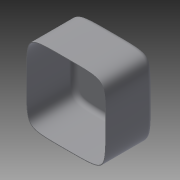
# Autodesk Inventor part: Base Plate
Saved by Autodesk Inventor 2014 SP1 (Build 180222100, 222)
## iProperties
Created: 2014-01-02
Part Number: Base Plate
Material: Generic
Document SubType Name: Modeling
Designer: tom
Density: 1 g/cm^3
Appearance: Default
Author: tom
Autodesk Inventor part; units mm, degrees
ref_plane "YZ Plane" through (0, 0, 0) normal (1, 0, 0) x (0, 1, 0)
ref_plane "XZ Plane" through (0, 0, 0) normal (0, 1, 0) x (-1, 0, 0)
ref_plane "XY Plane" through (0, 0, 0) normal (0, 0, 1) x (1, 0, 0)
sketch "Sketch1" plane through (0, 0, 0) normal (0, 0, 1) x (1, 0, 0)
  line L0 (-95.25, 72.009) -> (-95.25, 148.209) construction
  line L1 (-95.25, 148.209) -> (-95.25, 167.259) construction
  line L2 (-95.25, 167.259) -> (-76.2, 167.259) construction
  line L3 (-76.2, 167.259) -> (0, 167.259) construction
  spline S0 degree 4 poles (-95.25, 72.009) (-95.25, 148.209) (-95.25, 167.259) (-76.2, 167.259) (0, 167.259) knots 1 1 1 1 1 2 2 2 2 2
  line L4 (0, -23.241) -> (-76.2, -23.241) construction
  line L5 (-76.2, -23.241) -> (-95.25, -23.241) construction
  line L6 (-95.25, -23.241) -> (-95.25, -4.191) construction
  line L7 (-95.25, -4.191) -> (-95.25, 72.009) construction
  spline S1 degree 4 poles (0, -23.241) (-76.2, -23.241) (-95.25, -23.241) (-95.25, -4.191) (-95.25, 72.009) knots 1 1 1 1 1 2 2 2 2 2
  line L8 (95.25, 72.009) -> (95.25, -4.191) construction
  line L9 (95.25, -4.191) -> (95.25, -23.241) construction
  line L10 (95.25, -23.241) -> (76.2, -23.241) construction
  line L11 (76.2, -23.241) -> (0, -23.241) construction
  spline S2 degree 4 poles (95.25, 72.009) (95.25, -4.191) (95.25, -23.241) (76.2, -23.241) (0, -23.241) knots 1 1 1 1 1 2 2 2 2 2
  line L12 (0, 167.259) -> (76.2, 167.259) construction
  line L13 (76.2, 167.259) -> (95.25, 167.259) construction
  line L14 (95.25, 167.259) -> (95.25, 148.209) construction
  line L15 (95.25, 148.209) -> (95.25, 72.009) construction
  spline S3 degree 4 poles (0, 167.259) (76.2, 167.259) (95.25, 167.259) (95.25, 148.209) (95.25, 72.009) knots 1 1 1 1 1 2 2 2 2 2
  point P0 (0, 72.009)
  dimension "d12" = 76.2
  dimension "d13" = 76.2
  constraints: 12 other
  measures "d12" distance of L3.end L2.end
  measures "d13" distance of L0.start L0.end
extrude "Extrusion1" add sketch "Sketch1" along normal blind 114.3
fillet "Fillet1" radius 12.7 4 edges at (-84.5344, -12.5254, 0) (84.5344, -12.5254, 0) (84.5344, 156.5434, 0) (-84.5344, 156.5434, 0)
shell "Shell1" thickness 1.5875 removed faces 1 at (-31.75, 72.009, 114.3)
body "Solid1"
